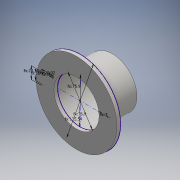
# Autodesk Inventor part: Fixture
Saved by Autodesk Inventor 2016 (Build 200138000, 138)
## iProperties
Created: 2015-07-19
Part Number: Fixture
Material: Generic
Document SubType Name: Modeling
Designer: bastli
Density: 1 g/cm^3
Appearance: Default
Author: bastli
Autodesk Inventor part; units mm, degrees
ref_plane "YZ Plane" through (0, 0, 0) normal (1, 0, 0) x (0, 1, 0)
ref_plane "XZ Plane" through (0, 0, 0) normal (0, 1, 0) x (-1, 0, 0)
ref_plane "XY Plane" through (0, 0, 0) normal (0, 0, 1) x (1, 0, 0)
sketch "Sketch1" plane through (0, 0, 0) normal (0, 1, 0) x (-1, 0, 0)
  circle A0 centre (0, 0) radius 67.77
  circle A1 centre (0, 0) radius 38.45
  circle A2 centre (0, 0) radius 41.45
  circle A3 centre (0, 0) radius 37.95
  line L0 (67.77, 0) -> (-67.77, 0) construction
  line L1 (0, 67.77) -> (0, -67.77) construction
  line L2 (62.61, -8) -> (46.61, -8) construction
  line L3 (46.61, -8) -> (46.61, 8) construction
  line L4 (46.61, 8) -> (62.61, 8) construction
  line L5 (62.61, 8) -> (62.61, -8) construction
  line L6 (62.61, -8) -> (46.61, 8) construction
  line L7 (46.61, -8) -> (62.61, 8) construction
  line L8 (64.77, -10.16) -> (44.45, -10.16) construction
  line L9 (44.45, -10.16) -> (44.45, 10.16) construction
  line L10 (44.45, 10.16) -> (64.77, 10.16) construction
  line L11 (64.77, 10.16) -> (64.77, -10.16) construction
  line L12 (64.77, -10.16) -> (44.45, 10.16) construction
  line L13 (44.45, -10.16) -> (64.77, 10.16) construction
  line L14 (64.77, 0) -> (67.77, 0) construction
  line L15 (44.45, 0) -> (41.45, 0) construction
  point P0 (54.61, 0)
  point P1 (-62.61, 8)
  point P2 (-46.61, 8)
  point P3 (-46.61, -8)
  point P4 (-62.61, -8)
  dimension "d0" = 135.54
  dimension "d1" = 76.9
  dimension "d2" = 3
  dimension "d3" = 75.9
  dimension "d4" = 16
  dimension "d5" = 16
  dimension "d6" = 20.32
  dimension "d7" = 20.32
  constraints: 32 end point, 9 midpoint, 7 coincident, 4 parallel, 4 point on circle, 4 symmetric about line, 3 centre point, 3 horizontal, 2 collinear, 2 perpendicular, 2 point on line, 1 horizontal alignment, 1 vertical, 2 other
  measures "d0" diameter of A0
  measures "d1" diameter of A1
  measures "d3" diameter of A3
  measures "d4" distance of L3.end L4.end
  measures "d5" distance of L4.end L2.start
  measures "d6" distance of L9.end L10.end
  measures "d7" distance of L10.end L8.start
extrude "Extrusion1" add sketch "Sketch1" against normal blind 6 contours A0 | A1 | A2
extrude "Extrusion2" add sketch "Sketch1" along normal blind 54 contours A2
equation "\"d0\" = outer_radius"
equation "\"d1\" = pvc_radius"
equation "\"d2\" = thickness"
equation "\"d3\" = pcv_foot_radius"
equation "\"d4\" = nema_8_hole_distance"
equation "\"d5\" = nema_8_hole_distance"
equation "\"d6\" = nema_8_width"
equation "\"d7\" = nema_8_width"
equation "\"d8\" = 2 * thickness"
equation "\"d10\" = fixture_height"
equation "\"thickness\" = 3"
equation "\"outer_radius\" = 6 * thickness + pvc_radius + 2 * nema_8_width"
equation "\"pvc_radius\" = 76.9"
equation "\"pcv_foot_radius\" = 75.9"
equation "\"nema_8_width\" = 20.32"
equation "\"nema_8_hole_distance\" = 16"
equation "\"fixture_height\" = 18 * thickness"
body "Solid1"
